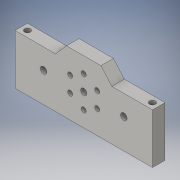
# Autodesk Inventor part: m_mount_r
Saved by Autodesk Inventor 2016 (Build 200138000, 138)
## iProperties
Created: 2016-12-01
Part Number: m_mount_r
Material: 一般
Document SubType Name: Modeling
Designer: KOTA-NPC2
Density: 1 g/cm^3
Appearance: 既定
Author: KOTA-NPC2
Autodesk Inventor part; units mm, degrees
ref_plane "YZ Plane" through (0, 0, 0) normal (1, 0, 0) x (0, 1, 0)
ref_plane "XZ Plane" through (0, 0, 0) normal (0, 1, 0) x (-1, 0, 0)
ref_plane "XY Plane" through (0, 0, 0) normal (0, 0, 1) x (1, 0, 0)
sketch "構築線" plane through (0, 0, 0) normal (0, 0, 1) x (1, 0, 0)
  circle A0 centre (0, 0) radius 8.5
  circle A1 centre (0, 0) radius 2.8 construction
  circle A2 centre (0, 0) radius 5 construction
  line L0 (0, -10) -> (-25, -10) construction
  line L1 (0, -13) -> (-25, -13) construction
  circle A3 centre (-12.8421, -0.45) radius 10.05 construction
  circle A4 centre (-12.8421, -0.45) radius 12.55 construction
  circle A5 centre (0, 5) radius 0.8
  circle A6 centre (-4.3301, 2.5) radius 0.8
  circle A7 centre (-4.3301, -2.5) radius 0.8
  circle A8 centre (0, -5) radius 0.8
  circle A9 centre (4.3301, -2.5) radius 0.8
  circle A10 centre (4.3301, 2.5) radius 0.8
  line L2 (25, -10) -> (0, -10) construction
  circle A11 centre (12.8421, -0.45) radius 10.05 construction
  circle A12 centre (12.8421, -0.45) radius 12.55 construction
  line L3 (0, -13) -> (25, -13) construction
  line L4 (-22, -10) -> (0, -10)
  line L5 (0, 25) -> (0, -25)
  line L6 (0, -10) -> (22, -10)
  circle A13 centre (0, 0) radius 3
  circle A14 centre (0, 0) radius 1
  circle A15 centre (12.8421, -0.45) radius 1.05
  circle A16 centre (-12.8421, -0.45) radius 1.05
  circle A17 centre (12.8421, -0.45) radius 2.75
  circle A18 centre (-12.8421, -0.45) radius 2.75
  line L7 (-22, 6) -> (-22, -10)
  line L8 (22, -10) -> (22, 6)
  line L9 (-22, 6) -> (-9, 6)
  line L10 (-9, 6) -> (-5.5, 10)
  line L11 (22, 6) -> (9, 6)
  line L12 (9, 6) -> (5.5, 10)
  line L13 (-5.5, 10) -> (5.5, 10)
  point P0 (-5.5355, 6.4504)
  point P1 (5.5355, 6.4504)
  dimension "d22" = 20.1
  dimension "d41" = 20.1
  dimension "d0" = 17
  dimension "d1" = 5.6
  dimension "d2" = 10
  dimension "d12" = 25
  dimension "d13" = 10
  dimension "d14" = 0
  dimension "d17" = 0
  dimension "d18" = 25
  dimension "d19" = 3
  dimension "d23" = 25.1
  dimension "d29" = 1.6
  dimension "d30" = 0
  dimension "d31" = 5
  dimension "d34" = 360
  dimension "d38" = 25
  dimension "d42" = 25.1
  dimension "d43" = 25
  dimension "d46" = 22
  dimension "d49" = 50
  dimension "d50" = 25
  dimension "d51" = 25
  dimension "d52" = 22
  dimension "d58" = 6
  dimension "d59" = 2
  dimension "d99" = 2.1
  dimension "d100" = 2.1
  dimension "d105" = 5.5
  dimension "d106" = 5.5
  dimension "d253" = 16
  dimension "d254" = 16
  dimension "d255" = 13
  dimension "d257" = 13
  dimension "d258" = 3.5
  dimension "d259" = 3.5
  dimension "d261" = 4
  constraints: 28 end point, 17 centre point, 8 coincident, 8 horizontal, 3 vertical, 2 point on circle, 2 tangent, 1 collinear, 1 concentric, 1 point on line, 23 other
  measures "d0" diameter of A0
  measures "d1" diameter of A1
  measures "d2" diameter of A2
  measures "d12" distance of L0.start L0.end
  measures "d13" distance from line of point (0, 0) L0
  measures "d14" horizontal distance of point (0, 0) L0.start
  measures "d17" horizontal distance of L1.start point (0, 0)
  measures "d18" distance of L1.start L1.end
  measures "d19" distance between parallel lines of L1 L0
  measures "d23" diameter of A4
  measures "d29" diameter of A5
  measures "d30" horizontal distance of point (0, 0) A5.centre
  measures "d31" distance of point (0, 0) A5.centre
  measures "d38" distance of L0.start L2.start
  measures "d42" diameter of A12
  measures "d43" distance of L1.start L3.end
  measures "d46" distance of L0.start L4.start
  measures "d49" distance of L5.start L5.end
  measures "d50" distance of point (0, 0) L5.start
  measures "d51" distance of L5.end point (0, 0)
  measures "d52" distance of L0.start L6.end
  measures "d58" diameter of A13
  measures "d59" diameter of A14
  measures "d99" diameter of A15
  measures "d100" diameter of A16
  measures "d105" diameter of A17
  measures "d106" diameter of A18
  measures "d253" distance of L7.start L4.start
  measures "d254" distance of L6.end L8.end
  measures "d255" distance of L7.start L9.end
  measures "d257" distance of L8.end L11.end
  measures "d258" horizontal distance of L10.end L9.end
  measures "d259" horizontal distance of L11.end L12.end
  measures "d261" distance between parallel lines of L13 L11
extrude "押し出し11" add sketch "構築線" along normal mid plane 4 contours A0 L5 A8 A13 A5 | A0 L5 L13 L12 L11 L8 L6 | L5 A5 A13 A8 A0 | A0 L5 L4 L7 L9 L10 L13 | A13 L5 A14 | L5 A14 A13 | A17 | A18
sketch "固定穴" plane through (0, 0, -2) normal (0, 0, -1) x (-1, 0, 0)
  circle A0 centre (0, 0) radius 8.5
  line L0 (0, -8.6) -> (-25, -8.6) construction
  line L1 (25, -8.6) -> (0, -8.6) construction
  line L2 (0, 25) -> (0, -25)
  circle A1 centre (12.8421, -0.45) radius 2.75
  circle A2 centre (-12.8421, -0.45) radius 2.75
  circle A3 centre (0, 0) radius 1 projected
  circle A4 centre (-12.8421, -0.45) radius 1.05 projected
  circle A5 centre (12.8421, -0.45) radius 1.05 projected
  circle A6 centre (0, 0) radius 3.05
  dimension "d180" = 17
  dimension "d183" = 25
  dimension "d195" = 25
  dimension "d200" = 50
  dimension "d208" = 5.5
  dimension "d209" = 5.5
  dimension "d216" = 6.1
  constraints: 6 end point, 4 centre point, 3 concentric, 2 horizontal, 2 vertical, 1 coincident, 1 collinear
  measures "d180" diameter of A0
  measures "d183" distance of L0.start L0.end
  measures "d195" distance of L0.start L1.start
  measures "d200" distance of L2.start L2.end
  measures "d208" diameter of A1
  measures "d209" diameter of A2
  measures "d216" diameter of A6
extrude "押し出し19" cut sketch "固定穴" against normal blind 2 contours A1 | A2 | A4 | A5
extrude "押し出し21" cut sketch "固定穴" against normal blind 2.1 contours A6 L2 A3 | L2 A3 A6
sketch "ねじ穴+固定(基板)" plane through (-22, -10, 2) normal (0, -1, 0) x (1, 0, 0)
  circle A0 centre (38, -2) radius 1
  line L0 (44, 0) -> (44, -4) projected
  line L1 (44, -2) -> (0, -2) construction
  line L2 (0, 0) -> (0, -4) projected
  circle A1 centre (6, -2) radius 1
  line L3 (34.8, -3) -> (32.8, -3)
  line L4 (32.8, -3) -> (32.8, -1)
  line L5 (32.8, -1) -> (34.8, -1)
  line L6 (34.8, -1) -> (34.8, -3)
  line L7 (34.8, -3) -> (32.8, -1) construction
  line L8 (32.8, -3) -> (34.8, -1) construction
  line L9 (11.2, -1) -> (9.2, -1)
  line L10 (9.2, -1) -> (9.2, -3)
  line L11 (9.2, -3) -> (11.2, -3)
  line L12 (11.2, -3) -> (11.2, -1)
  line L13 (11.2, -1) -> (9.2, -3) construction
  line L14 (9.2, -1) -> (11.2, -3) construction
  point P0 (22, -2)
  point P1 (33.8, -2)
  point P2 (33.8, -2)
  point P3 (10.2, -2)
  point P4 (10.2, -2)
  dimension "d219" = 2
  dimension "d220" = 6
  dimension "d221" = 6
  dimension "d222" = 2
  dimension "d223" = 2
  dimension "d224" = 2
  dimension "d225" = 4.2
  dimension "d226" = 2
  dimension "d227" = 2
  dimension "d228" = 4.2
  constraints: 26 end point, 8 midpoint, 4 parallel, 4 point on line, 2 centre point, 2 horizontal, 2 perpendicular
  measures "d219" diameter of A0
  measures "d220" distance from line of L0 A0.centre
  measures "d221" distance from line of L2 A1.centre
  measures "d222" diameter of A1
  measures "d223" distance of L3.start L3.end
  measures "d224" distance of L3.end L4.end
  measures "d225" distance of A0.centre point (33.8, -2)
  measures "d226" distance of L11.end L10.end
  measures "d227" distance of L10.end L9.end
  measures "d228" distance of A1.centre point (10.2, -2)
hole "ねじ穴(基板)" at (16, -10, 0) at (-16, -10, 0) direction (0, 1, 0) diameter 1.6 depth 3.5 tip angle 118
extrude "押し出し22" add sketch "ねじ穴+固定(基板)" along normal blind 1 contours L3 L4 L5 L6 | L12 L11 L10 L9
fillet "フィレット1" radius 0.5 4 edges at (12.8, -10.5, -1) (12.8, -10.5, 1) (10.8, -10.5, -1) (10.8, -10.5, 1)
fillet "フィレット2" radius 0.5 4 edges at (-12.8, -10.5, -1) (-12.8, -10.5, 1) (-10.8, -10.5, -1) (-10.8, -10.5, 1)
sketch "スケッチ20" plane through (-22, 6, 2) normal (0, 1, 0) x (1, 0, 0)
  line L0 (0, 0) -> (0, 4) projected
  line L1 (13, 0) -> (0, 0) projected
  line L2 (13, 0) -> (13, 4) projected
  line L3 (0, 4) -> (13, 4) projected
  line L4 (31, 0) -> (31, 4) projected
  line L5 (44, 0) -> (31, 0) projected
  line L6 (44, 0) -> (44, 4) projected
  line L7 (31, 4) -> (44, 4) projected
  line L8 (0, 0) -> (4, 0) construction
  line L9 (4, 0) -> (4, 4) construction
  line L10 (4, 4) -> (0, 4) construction
  line L11 (0, 4) -> (0, 0) construction
  line L12 (44, 0) -> (40, 0) construction
  line L13 (40, 0) -> (40, 4) construction
  line L14 (40, 4) -> (44, 4) construction
  line L15 (44, 4) -> (44, 0) construction
  line L16 (4, 0) -> (0, 4) construction
  line L17 (0, 0) -> (4, 4) construction
  line L18 (40, 0) -> (44, 4) construction
  line L19 (44, 0) -> (44, 4) construction
  line L20 (44, 0) -> (40, 4) construction
  circle A0 centre (2, 2) radius 0.95
  circle A1 centre (42, 2) radius 0.95
  point P0 (22, 2)
  dimension "d290" = 4
  dimension "d291" = 4
  dimension "d292" = 4
  dimension "d293" = 4
  dimension "d294" = 1.9
  dimension "d295" = 1.9
  constraints: 24 end point, 4 parallel, 2 centre point, 2 horizontal, 2 midpoint, 2 perpendicular
  measures "d290" distance of L10.end L9.end
  measures "d291" distance of L9.end L8.end
  measures "d292" distance of L13.end L14.end
  measures "d293" distance of L12.end L13.end
  measures "d294" diameter of A0
  measures "d295" diameter of A1
extrude "押し出し28" cut sketch "スケッチ20" against normal blind 3.5 contours A0 | A1
sketch "外形側面（dxf出力用）" plane through (0, 0, 2) normal (0, 0, 1) x (1, 0, 0)
  line L0 (-10, 6) -> (-5.5, 10)
  line L1 (-5.5, 10) -> (-10, 6)
  line L2 (-10, 6) -> (-22, 6)
  line L3 (-22, 6) -> (-22, -11)
  line L4 (-22, -11) -> (22, -11)
  line L5 (22, -11) -> (22, 6)
  line L6 (22, 6) -> (10, 6) projected
  line L7 (5.5, 10) -> (-5.5, 10) projected
  line L8 (10, 6) -> (5.5, 10)
  line L9 (5.5, 10) -> (-5.5, 10)
  line L10 (22, 6) -> (10, 6)
  circle A0 centre (0, 0) radius 2.8 projected
  circle A1 centre (4.3301, 2.5) radius 0.8 projected
  circle A2 centre (4.3301, -2.5) radius 0.8 projected
  circle A3 centre (0, -5) radius 0.8 projected
  circle A4 centre (-4.3301, -2.5) radius 0.8 projected
  circle A5 centre (-4.3301, 2.5) radius 0.8 projected
  circle A6 centre (0, 5) radius 0.8 projected
  circle A7 centre (0, 0) radius 8.5 projected
  circle A8 centre (0, 0) radius 1 projected
  circle A9 centre (-12.8421, -0.45) radius 1.05 projected
  circle A10 centre (-12.8421, -0.45) radius 2.75 projected
  circle A11 centre (12.8421, -0.45) radius 1.05 projected
  circle A12 centre (12.8421, -0.45) radius 2.75 projected
  constraints: 24 end point, 1 collinear, 1 horizontal, 1 perpendicular, 1 vertical
sketch "外形底面（dxf出力用）" plane through (-22, -10, 2) normal (0, -1, 0) x (1, 0, 0)
  arc A0 (11.2, -1.5) -> (10.7, -1) centre (10.7, -1.5) ccw projected
  line L0 (10.7, -1) -> (9.7, -1) projected
  arc A1 (9.7, -1) -> (9.2, -1.5) centre (9.7, -1.5) ccw projected
  line L1 (9.2, -1.5) -> (9.2, -2.5) projected
  arc A2 (9.2, -2.5) -> (9.7, -3) centre (9.7, -2.5) ccw projected
  line L2 (9.7, -3) -> (10.7, -3) projected
  arc A3 (10.7, -3) -> (11.2, -2.5) centre (10.7, -2.5) ccw projected
  line L3 (11.2, -2.5) -> (11.2, -1.5) projected
  arc A4 (33.3, -1) -> (32.8, -1.5) centre (33.3, -1.5) ccw projected
  line L4 (32.8, -1.5) -> (32.8, -2.5) projected
  arc A5 (32.8, -2.5) -> (33.3, -3) centre (33.3, -2.5) ccw projected
  line L5 (33.3, -3) -> (34.3, -3) projected
  arc A6 (34.3, -3) -> (34.8, -2.5) centre (34.3, -2.5) ccw projected
  line L6 (34.8, -2.5) -> (34.8, -1.5) projected
  arc A7 (34.8, -1.5) -> (34.3, -1) centre (34.3, -1.5) ccw projected
  line L7 (34.3, -1) -> (33.3, -1) projected
  circle A8 centre (38, -2) radius 0.8 projected
  circle A9 centre (6, -2) radius 0.8 projected
  line L8 (31, -4) -> (44, -4) projected
  line L9 (0, -4) -> (13, -4) projected
  line L10 (13, 0) -> (0, 0) projected
  line L11 (44, 0) -> (31, 0) projected
  line L12 (0, 0) -> (0, -4) projected
  line L13 (44, 0) -> (44, -4) projected
  line L14 (31, 0) -> (31, -4) projected
  line L15 (31, -4) -> (31, 0)
  line L16 (31, 0) -> (13, 0)
  line L17 (13, 0) -> (13, -4) projected
  line L18 (13, 0) -> (13, -4)
  line L19 (13, -4) -> (31, -4)
  point P0 (22, -2)
  constraints: 8 end point, 2 perpendicular, 2 vertical
sketch "外形上面(dxf出力用)" plane through (-22, 6, 2) normal (0, 1, 0) x (1, 0, 0)
  line L0 (44, 4) -> (0, 4) projected
  line L1 (44, 0) -> (44, 4) projected
  line L2 (0, 0) -> (44, 0) projected
  line L3 (0, 0) -> (0, 4) projected
  circle A0 centre (2, 2) radius 0.95 projected
  circle A1 centre (42, 2) radius 0.95 projected
  point P0 (22, 2)
  point P1 (13, 4)
sketch "スケッチ25" plane through (0, 0, -2) normal (0, 0, -1) x (-1, 0, 0)
  circle A0 centre (-12.8421, -0.45) radius 1.05 projected
  circle A1 centre (0, 0) radius 1 projected
  circle A2 centre (12.8421, -0.45) radius 1.05 projected
  line L0 (12.3, -11) -> (11.3, -11) projected
  line L1 (-11.3, -11) -> (-12.3, -11) projected
  line L2 (5.5, 10) -> (-5.5, 10) projected
  line L3 (-5.5, 10) -> (-9, 6) projected
  line L4 (-9, 6) -> (-22, 6) projected
  line L5 (-22, 6) -> (-22, -10) projected
  line L6 (9, 6) -> (5.5, 10) projected
  line L7 (22, 6) -> (9, 6) projected
  line L8 (22, -10) -> (22, 6) projected
  circle A3 centre (0, 5) radius 0.8 projected
  circle A4 centre (-4.3301, 2.5) radius 0.8 projected
  circle A5 centre (-4.3301, -2.5) radius 0.8 projected
  circle A6 centre (0, -5) radius 0.8 projected
  circle A7 centre (4.3301, -2.5) radius 0.8 projected
  circle A8 centre (4.3301, 2.5) radius 0.8 projected
  line L9 (-22, -10) -> (-22, -11)
  line L10 (-22, -11) -> (-12.3, -11)
  line L11 (-11.3, -11) -> (11.3, -11)
  line L12 (12.3, -11) -> (22, -11)
  line L13 (22, -11) -> (22, -10)
  circle A9 centre (12.8421, -0.45) radius 2.75 projected
  circle A10 centre (-12.8421, -0.45) radius 2.75 projected
  circle A11 centre (0, 0) radius 3.05 projected
  constraints: 10 end point, 2 perpendicular, 1 collinear, 1 point on line, 1 vertical
sketch "冶具" plane through (0, 0, 2) normal (0, 0, 1) x (1, 0, 0)
  line L0 (-19, 6) -> (-9, 6)
  line L1 (-5.5, 10) -> (5.5, 10)
  line L2 (9, 6) -> (19, 6)
  line L3 (-11.3, -11) -> (-12.3, -11) construction
  line L4 (12.3, -11) -> (11.3, -11) construction
  line L5 (22, 6) -> (22, -11)
  line L6 (-22, 6) -> (-22, -11)
  line L7 (-19, -11) -> (19, -11)
  line L8 (-22, 6) -> (-22, 7.5)
  line L9 (-22, 7.5) -> (-19, 7.5)
  line L10 (-19, 7.5) -> (-19, 6)
  line L11 (-5.5, 10) -> (-7, 10)
  line L12 (-7, 10) -> (-7, 8.2857)
  line L13 (-7, 8.2857) -> (-9, 6)
  line L14 (-5.5, 10) -> (5.5, 10) projected
  line L15 (5.5, 10) -> (7, 10)
  line L16 (7, 10) -> (7, 8.2857)
  line L17 (7, 8.2857) -> (9, 6)
  line L18 (19, -11) -> (19, -12.5)
  line L19 (19, -12.5) -> (22, -12.5)
  line L20 (22, -12.5) -> (22, -11)
  line L21 (-22, -11) -> (-22, -12.5)
  line L22 (-22, -12.5) -> (-19, -12.5)
  line L23 (-19, -12.5) -> (-19, -11)
  line L24 (22, 6) -> (22, 7.5)
  line L25 (22, 7.5) -> (19, 7.5)
  line L26 (19, 7.5) -> (19, 6)
  point P0 (0, 0)
  dimension "d310" = 3
  dimension "d311" = 3
  dimension "d316" = 1.5
  dimension "d317" = 1.5
  dimension "d318" = 1.5
  dimension "d319" = 1.5
  dimension "d320" = 38
  dimension "d321" = 17
  dimension "d322" = 17
  dimension "d323" = 11
  dimension "d324" = 10
  dimension "d325" = 10
  dimension "d326" = 3
  dimension "d327" = 3
  dimension "d328" = 2
  dimension "d329" = 2
  dimension "d330" = 1.5
  dimension "d331" = 1.5
  constraints: 50 end point, 9 perpendicular, 4 vertical, 3 horizontal, 3 point on line
  measures "d310" distance of L5.end L7.end
  measures "d311" distance of L6.end L7.start
  measures "d316" distance of L7.end L18.end
  measures "d317" distance of L6.end L21.end
  measures "d318" distance of L5.start L24.end
  measures "d319" distance of L6.start L8.end
  measures "d320" distance of L7.start L7.end
  measures "d321" distance of L6.start L6.end
  measures "d322" distance of L5.start L5.end
  measures "d323" distance of L1.start L1.end
  measures "d324" distance of L0.start L0.end
  measures "d325" distance of L2.start L2.end
  measures "d326" distance of L24.end L25.end
  measures "d327" distance of L8.end L9.end
  measures "d328" horizontal distance of L12.end L13.end
  measures "d329" horizontal distance of L16.end L2.start
  measures "d330" distance of L1.end L15.end
  measures "d331" distance of L1.start L11.end
sketch "スケッチ27" plane through (-22, -10, 2) normal (0, -1, 0) x (1, 0, 0)
  line L0 (32.8, -2.5) -> (32.8, -1.5) construction
  arc A0 (33.3, -1) -> (32.8, -1.5) centre (33.3, -1.5) ccw construction
  line L1 (33.3, -1) -> (34.3, -1) construction
  arc A1 (34.8, -1.5) -> (34.3, -1) centre (34.3, -1.5) ccw construction
  line L2 (34.8, -1.5) -> (34.8, -2.5) construction
  arc A2 (34.3, -3) -> (34.8, -2.5) centre (34.3, -2.5) ccw construction
  line L3 (34.3, -3) -> (33.3, -3) construction
  arc A3 (32.8, -2.5) -> (33.3, -3) centre (33.3, -2.5) ccw construction
  line L4 (11.2, -1.5) -> (11.2, -2.5) construction
  arc A4 (10.7, -3) -> (11.2, -2.5) centre (10.7, -2.5) ccw construction
  line L5 (10.7, -3) -> (9.7, -3) construction
  arc A5 (9.2, -2.5) -> (9.7, -3) centre (9.7, -2.5) ccw construction
  line L6 (9.2, -2.5) -> (9.2, -1.5) construction
  arc A6 (9.7, -1) -> (9.2, -1.5) centre (9.7, -1.5) ccw construction
  line L7 (9.7, -1) -> (10.7, -1) construction
  arc A7 (11.2, -1.5) -> (10.7, -1) centre (10.7, -1.5) ccw construction
  circle A8 centre (38, -2) radius 0.8 construction
  circle A9 centre (6, -2) radius 0.8 construction
  line L8 (44, 0) -> (44, -4) construction
  line L9 (0, 0) -> (44, 0) construction
  line L10 (0, 0) -> (0, -4) construction
  line L11 (44, -4) -> (0, -4) construction
  line L12 (0, 0) -> (0, 1.5)
  line L13 (0, 1.5) -> (3, 1.5)
  line L14 (3, 1.5) -> (3, 0)
  line L15 (3, 0) -> (41, 0)
  line L16 (0, 0) -> (44, 0) projected
  line L17 (44, 0) -> (44, 1.5)
  line L18 (44, 1.5) -> (41, 1.5)
  line L19 (41, 1.5) -> (41, 0)
  line L20 (0, -4) -> (0, -5.5)
  line L21 (0, -5.5) -> (3, -5.5)
  line L22 (3, -5.5) -> (3, -4)
  line L23 (44, -4) -> (44, -5.5)
  line L24 (44, -5.5) -> (41, -5.5)
  line L25 (41, -5.5) -> (41, -4)
  line L26 (41, -4) -> (3, -4)
  line L27 (44, 0) -> (44, -4)
  line L28 (0, 0) -> (0, -4)
  circle A10 centre (42, -2) radius 0.95 projected
  circle A11 centre (2, -2) radius 0.95 projected
  point P0 (22, -2)
  dimension "d332" = 1.5
  dimension "d333" = 3
  dimension "d334" = 1.5
  dimension "d335" = 3
  dimension "d336" = 1.5
  dimension "d337" = 3
  dimension "d338" = 1.5
  dimension "d339" = 3
  constraints: 32 end point, 7 perpendicular, 6 vertical, 4 point on line, 1 collinear, 1 horizontal
  measures "d332" distance of L9.start L12.end
  measures "d333" distance of L12.end L13.end
  measures "d334" distance of L8.start L17.end
  measures "d335" distance of L17.end L18.end
  measures "d336" distance of L10.end L20.end
  measures "d337" distance of L20.end L21.end
  measures "d338" distance of L8.end L23.end
  measures "d339" distance of L23.end L24.end
sketch "スケッチ28" plane through (-5.5, 10, 2) normal (0, 1, 0) x (1, 0, 0)
  line L0 (14.5, 0) -> (14.5, 4) projected
  line L1 (-3.5, 0) -> (-3.5, 4) projected
  line L2 (-3.5, 4) -> (-3.5, 5.5)
  line L3 (-3.5, 5.5) -> (-0.5, 5.5)
  line L4 (-0.5, 5.5) -> (-0.5, 4)
  line L5 (-3.5, 0) -> (-3.5, -1.5)
  line L6 (-3.5, -1.5) -> (-0.5, -1.5)
  line L7 (-0.5, -1.5) -> (-0.5, 0)
  line L8 (14.5, 4) -> (14.5, 5.5)
  line L9 (14.5, 5.5) -> (11.5, 5.5)
  line L10 (11.5, 5.5) -> (11.5, 4)
  line L11 (14.5, 0) -> (14.5, -1.5)
  line L12 (14.5, -1.5) -> (11.5, -1.5)
  line L13 (11.5, -1.5) -> (11.5, 0)
  line L14 (11.5, 0) -> (-0.5, 0)
  line L15 (-0.5, 4) -> (11.5, 4)
  circle A0 centre (21.5, 2) radius 0.8 projected
  circle A1 centre (-10.5, 2) radius 0.8 projected
  line L16 (17.8, 1) -> (16.8, 1) projected
  arc A2 (17.8, 1) -> (18.3, 1.5) centre (17.8, 1.5) ccw projected
  line L17 (18.3, 2.5) -> (18.3, 1.5) projected
  arc A3 (18.3, 2.5) -> (17.8, 3) centre (17.8, 2.5) ccw projected
  line L18 (16.8, 3) -> (17.8, 3) projected
  arc A4 (16.8, 3) -> (16.3, 2.5) centre (16.8, 2.5) ccw projected
  line L19 (16.3, 1.5) -> (16.3, 2.5) projected
  arc A5 (16.3, 1.5) -> (16.8, 1) centre (16.8, 1.5) ccw projected
  line L20 (-5.8, 1) -> (-6.8, 1) projected
  arc A6 (-5.8, 1) -> (-5.3, 1.5) centre (-5.8, 1.5) ccw projected
  line L21 (-5.3, 2.5) -> (-5.3, 1.5) projected
  arc A7 (-5.3, 2.5) -> (-5.8, 3) centre (-5.8, 2.5) ccw projected
  line L22 (-6.8, 3) -> (-5.8, 3) projected
  arc A8 (-6.8, 3) -> (-7.3, 2.5) centre (-6.8, 2.5) ccw projected
  line L23 (-7.3, 1.5) -> (-7.3, 2.5) projected
  arc A9 (-7.3, 1.5) -> (-6.8, 1) centre (-6.8, 1.5) ccw projected
  point P0 (5.5, 2)
  dimension "d340" = 1.5
  dimension "d341" = 3
  dimension "d342" = 1.5
  dimension "d343" = 3
  dimension "d344" = 1.5
  dimension "d345" = 3
  dimension "d346" = 1.5
  dimension "d347" = 3
  constraints: 28 end point, 7 perpendicular, 5 vertical, 1 horizontal, 1 parallel
  measures "d340" distance of L1.end L2.end
  measures "d341" distance of L2.end L3.end
  measures "d342" distance of L1.start L5.end
  measures "d343" distance of L5.end L6.end
  measures "d344" distance of L0.end L8.end
  measures "d345" distance of L8.end L9.end
  measures "d346" distance of L0.start L11.end
  measures "d347" distance of L11.end L12.end
equation "\"d18\" = d12"
